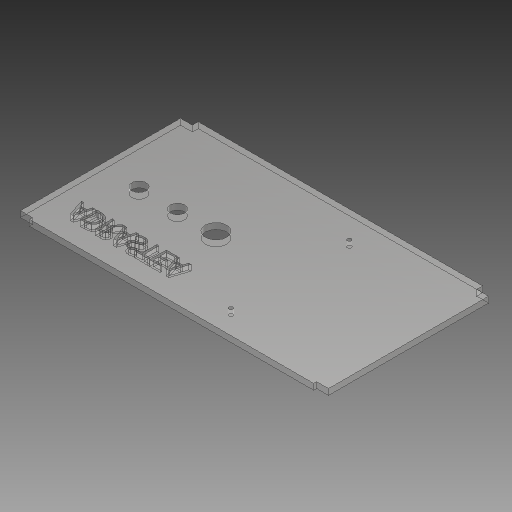
# Autodesk Inventor part: SeitenOben
Saved by Autodesk Inventor 2019 (Build 230136000, 136)
## iProperties
Created: 2018-04-27
Part Number: SeitenOben
Material: Polycarbonate, Clear
Document SubType Name: Modeling
Designer: Phil Erle
Density: 1.2 g/cm^3
Appearance: Polycarbonate - Clear
Author: Phil Erle
Autodesk Inventor part; units mm, degrees
ref_plane "YZ Plane" through (0, 0, 0) normal (1, 0, 0) x (0, 1, 0)
ref_plane "XZ Plane" through (0, 0, 0) normal (0, 1, 0) x (-1, 0, 0)
ref_plane "XY Plane" through (0, 0, 0) normal (0, 0, 1) x (1, 0, 0)
sketch "Sketch1" plane through (0, 0, 0) normal (0, 0, 1) x (1, 0, 0)
  line L0 (-130, 67.5) -> (-130, -67.5)
  line L1 (-130, -67.5) -> (-120, -67.5)
  line L2 (-120, -67.5) -> (-120, -70)
  line L3 (-120, -70) -> (120, -70)
  line L4 (120, -70) -> (120, -67.5)
  line L5 (120, -67.5) -> (130, -67.5)
  line L6 (130, -67.5) -> (130, 67.5)
  line L7 (130, 67.5) -> (120, 67.5)
  line L8 (120, 67.5) -> (120, 72.5)
  line L9 (120, 72.5) -> (-120, 72.5)
  line L10 (-120, 72.5) -> (-120, 67.5)
  line L11 (-130, 67.5) -> (-120, 67.5)
  point P0 (0, 0)
  point P1 (0, 72.5)
  point P2 (130, 0)
  point P3 (-130, 0)
  dimension "d0" = 5
  dimension "d1" = 240
  dimension "d2" = 10
  dimension "d3" = 10
  dimension "d4" = 2.5
  dimension "d5" = 135
  constraints: 24 end point, 8 perpendicular, 7 point on line, 3 midpoint, 1 horizontal alignment, 1 vertical, 1 vertical alignment
  measures "d0" distance of L7.end L8.end
  measures "d1" distance of L8.end L9.end
  measures "d2" distance of L0.start L10.end
  measures "d3" distance of L6.end L7.end
  measures "d4" distance of L3.end L4.end
  measures "d5" distance between parallel lines of L1 L11
extrude "Extrusion1" add sketch "Sketch1" along normal blind 5
sketch "Sketch2" plane through (0, 0, 5) normal (0, 0, 1) x (1, 0, 0)
  point P0 (0, 0)
  point P1 (-65, 0)
  point P2 (-32.5, 0)
  point P3 (-97.5, 0)
  dimension "d8" = 32.5
  dimension "d9" = 32.5
  dimension "d10" = 32.5
  constraints: 3 horizontal alignment
  measures "d8" distance of point (-65, 0) point (-32.5, 0)
  measures "d9" distance of point (0, 0) point (-32.5, 0)
  measures "d10" distance of point (-65, 0) point (-97.5, 0)
hole "Hole1" at (-65, 0, 5) at (-97.5, 0, 5) direction (0, 0, -1) diameter 12 depth 8 tip angle 118
sketch "Sketch3" plane through (0, 0, 5) normal (0, 0, 1) x (1, 0, 0)
  line L0 (30, 50) -> (30, -50) construction
  point P0 (0, 0)
  point P1 (30, 0)
  dimension "d18" = 100
  dimension "d19" = 30
  constraints: 2 coincident, 2 end point, 1 horizontal alignment, 1 midpoint, 1 vertical
  measures "d18" distance of L0.start L0.end
  measures "d19" distance of point (30, 0) point (0, 0)
hole "Hole2" at (30, 50, 5) at (30, -50, 5) direction (0, 0, -1) diameter 3.4 depth 8 tip angle 118 clearance for "Countersunk Flat Head Screw DIN EN ISO 2009" size "M3" standard "DIN"
sketch "Sketch5" plane through (0, 0, 0) normal (0, 0, -1) x (-1, 0, 0)
  line L0 (111.2571, -49) -> (18.7429, -49) construction
  line L1 (18.7429, -49) -> (18.7429, -35) construction
  line L2 (18.7429, -35) -> (111.2571, -35) construction
  line L3 (111.2571, -35) -> (111.2571, -49) construction
  circle A0 centre (65, 0) radius 6 projected
  line L4 (111.3478, -34.7504) -> (106.6282, -48.7504)
  line L5 (106.6282, -48.7504) -> (104.3365, -48.7504)
  line L6 (104.3365, -48.7504) -> (99.6169, -34.7504)
  line L7 (99.6169, -34.7504) -> (101.5796, -34.7504)
  line L8 (101.5796, -34.7504) -> (102.8503, -38.6645)
  line L9 (102.8503, -38.6645) -> (108.1939, -38.6645)
  line L10 (108.1939, -38.6645) -> (109.4645, -34.7504)
  line L11 (109.4645, -34.7504) -> (111.3478, -34.7504)
  line L12 (103.3608, -40.2528) -> (105.5277, -46.8444)
  line L13 (105.5277, -46.8444) -> (107.6833, -40.2528)
  line L14 (107.6833, -40.2528) -> (103.3608, -40.2528)
  spline S0 degree 2 poles (87.2506, -41.7391) (87.2506, -39.8217) (88.8049, -36.7358) (90.1096, -35.8736) knots 0 0 0 1 2 2 2
  spline S1 degree 2 poles (90.1096, -35.8736) (91.176, -35.2042) (93.3657, -34.7504) (95.0675, -34.7504) knots 0 0 0 1 2 2 2
  line L15 (95.0675, -34.7504) -> (98.2895, -34.7504)
  line L16 (98.2895, -34.7504) -> (98.2895, -48.7504)
  line L17 (98.2895, -48.7504) -> (95.1015, -48.7504)
  spline S2 degree 2 poles (95.1015, -48.7504) (93.1274, -48.7504) (90.8811, -48.1605) (90.0869, -47.6386) knots 0 0 0 1 2 2 2
  spline S3 degree 2 poles (90.0869, -47.6386) (88.7368, -46.7423) (87.2506, -43.7812) (87.2506, -41.7391) knots 0 0 0 1 2 2 2
  spline S4 degree 2 poles (89.1906, -41.7617) (89.1906, -43.3728) (90.2571, -45.6532) (91.3122, -46.2998) knots 0 0 0 1 2 2 2
  spline S5 degree 2 poles (91.3122, -46.2998) (92.061, -46.7423) (93.7514, -47.1394) (95.0107, -47.1394) knots 0 0 0 1 2 2 2
  line L18 (95.0107, -47.1394) -> (96.4289, -47.1394)
  line L19 (96.4289, -47.1394) -> (96.4289, -36.3614)
  line L20 (96.4289, -36.3614) -> (95.0107, -36.3614)
  spline S6 degree 2 poles (95.0107, -36.3614) (93.7741, -36.3614) (91.9021, -36.7585) (91.142, -37.2917) knots 0 0 0 1 2 2 2
  spline S7 degree 2 poles (91.142, -37.2917) (90.1663, -37.9498) (89.1906, -40.128) (89.1906, -41.7617) knots 0 0 0 1 2 2 2
  line L21 (74.3965, -34.7504) -> (76.813, -34.7504)
  line L22 (76.813, -34.7504) -> (81.2376, -40.3209)
  line L23 (81.2376, -40.3209) -> (83.3705, -40.3209)
  line L24 (83.3705, -40.3209) -> (83.3705, -34.7504)
  line L25 (83.3705, -34.7504) -> (85.2311, -34.7504)
  line L26 (85.2311, -34.7504) -> (85.2311, -48.7504)
  line L27 (85.2311, -48.7504) -> (81.6234, -48.7504)
  spline S8 degree 2 poles (81.6234, -48.7504) (80.4208, -48.7504) (78.7984, -48.4895) (78.061, -48.013) knots 0 0 0 1 2 2 2
  spline S9 degree 2 poles (78.061, -48.013) (77.3235, -47.5365) (76.4726, -46.0502) (76.4726, -44.9498) knots 0 0 0 1 2 2 2
  spline S10 degree 2 poles (76.4726, -44.9498) (76.4726, -43.4182) (78.0383, -41.342) (79.377, -40.8428) knots 0 0 0 1 2 2 2
  line L28 (79.377, -40.8428) -> (74.3965, -34.7504)
  spline S11 degree 2 poles (78.4127, -44.8023) (78.4127, -45.4149) (78.8438, -46.3566) (79.2976, -46.6629) knots 0 0 0 1 2 2 2
  spline S12 degree 2 poles (79.2976, -46.6629) (79.6947, -46.9238) (80.7498, -47.1394) (81.5213, -47.1394) knots 0 0 0 1 2 2 2
  line L29 (81.5213, -47.1394) -> (83.3705, -47.1394)
  line L30 (83.3705, -47.1394) -> (83.3705, -41.8752)
  line L31 (83.3705, -41.8752) -> (81.7368, -41.8752)
  spline S13 degree 2 poles (81.7368, -41.8752) (80.9313, -41.8752) (79.6493, -42.1588) (79.2068, -42.6013) knots 0 0 0 1 2 2 2
  spline S14 degree 2 poles (79.2068, -42.6013) (78.7984, -42.987) (78.4127, -44.0762) (78.4127, -44.8023) knots 0 0 0 1 2 2 2
  line L32 (74.7935, -34.7504) -> (70.0739, -48.7504)
  line L33 (70.0739, -48.7504) -> (67.7822, -48.7504)
  line L34 (67.7822, -48.7504) -> (63.0626, -34.7504)
  line L35 (63.0626, -34.7504) -> (65.0253, -34.7504)
  line L36 (65.0253, -34.7504) -> (66.296, -38.6645)
  line L37 (66.296, -38.6645) -> (71.6396, -38.6645)
  line L38 (71.6396, -38.6645) -> (72.9102, -34.7504)
  line L39 (72.9102, -34.7504) -> (74.7935, -34.7504)
  line L40 (66.8065, -40.2528) -> (68.9735, -46.8444)
  line L41 (68.9735, -46.8444) -> (71.129, -40.2528)
  line L42 (71.129, -40.2528) -> (66.8065, -40.2528)
  spline S15 degree 2 poles (57.8324, -34.5008) (59.3527, -34.5008) (61.4856, -35.1361) (62.4273, -35.59) knots 0 0 0 1 2 2 2
  line L43 (62.4273, -35.59) -> (62.4273, -37.9271)
  line L44 (62.4273, -37.9271) -> (62.2911, -37.9271)
  spline S16 degree 2 poles (62.2911, -37.9271) (61.3722, -37.0648) (59.0464, -36.1118) (57.9686, -36.1118) knots 0 0 0 1 2 2 2
  spline S17 degree 2 poles (57.9686, -36.1118) (56.4256, -36.1118) (54.8487, -37.3938) (54.8487, -38.4489) knots 0 0 0 1 2 2 2
  spline S18 degree 2 poles (54.8487, -38.4489) (54.8487, -39.2885) (55.6769, -40.3323) (56.5731, -40.5932) knots 0 0 0 1 2 2 2
  spline S19 degree 2 poles (56.5731, -40.5932) (57.2198, -40.7747) (58.2976, -41.0243) (59.1031, -41.2285) knots 0 0 0 1 2 2 2
  spline S20 degree 2 poles (59.1031, -41.2285) (59.8292, -41.4214) (60.9751, -42) (61.4175, -42.4652) knots 0 0 0 1 2 2 2
  spline S21 degree 2 poles (61.4175, -42.4652) (61.8487, -42.9303) (62.3252, -44.1783) (62.3252, -44.9951) knots 0 0 0 1 2 2 2
  spline S22 degree 2 poles (62.3252, -44.9951) (62.3252, -46.6969) (59.6704, -49) (57.6169, -49) knots 0 0 0 1 2 2 2
  spline S23 degree 2 poles (57.6169, -49) (56.437, -49) (54.3495, -48.5348) (53.4532, -48.0924) knots 0 0 0 1 2 2 2
  line L45 (53.4532, -48.0924) -> (53.4532, -45.8687)
  line L46 (53.4532, -45.8687) -> (53.5893, -45.8687)
  spline S24 degree 2 poles (53.5893, -45.8687) (54.2587, -46.4814) (56.3462, -47.389) (57.4921, -47.389) knots 0 0 0 1 2 2 2
  spline S25 degree 2 poles (57.4921, -47.389) (58.7854, -47.389) (60.3851, -46.175) (60.3851, -45.188) knots 0 0 0 1 2 2 2
  spline S26 degree 2 poles (60.3851, -45.188) (60.3851, -44.3031) (59.4435, -43.248) (58.5585, -43.0097) knots 0 0 0 1 2 2 2
  spline S27 degree 2 poles (58.5585, -43.0097) (57.9686, -42.8509) (56.2555, -42.4425) (55.6882, -42.2723) knots 0 0 0 1 2 2 2
  spline S28 degree 2 poles (55.6882, -42.2723) (54.2474, -41.8298) (52.9086, -40.0486) (52.9086, -38.7439) knots 0 0 0 1 2 2 2
  spline S29 degree 2 poles (52.9086, -38.7439) (52.9086, -37.9157) (53.578, -36.3274) (54.1793, -35.7715) knots 0 0 0 1 2 2 2
  spline S30 degree 2 poles (54.1793, -35.7715) (54.8487, -35.1588) (56.5504, -34.5008) (57.8324, -34.5008) knots 0 0 0 1 2 2 2
  line L47 (47.7465, -34.7504) -> (47.7465, -47.094)
  line L48 (47.7465, -47.094) -> (52.4435, -47.094)
  line L49 (52.4435, -47.094) -> (52.4435, -48.7504)
  line L50 (52.4435, -48.7504) -> (41.189, -48.7504)
  line L51 (41.189, -48.7504) -> (41.189, -47.094)
  line L52 (41.189, -47.094) -> (45.8859, -47.094)
  line L53 (45.8859, -47.094) -> (45.8859, -34.7504)
  line L54 (45.8859, -34.7504) -> (47.7465, -34.7504)
  line L55 (39.7709, -34.7504) -> (39.7709, -48.7504)
  line L56 (39.7709, -48.7504) -> (31.0123, -48.7504)
  line L57 (31.0123, -48.7504) -> (31.0123, -47.094)
  line L58 (31.0123, -47.094) -> (37.9102, -47.094)
  line L59 (37.9102, -47.094) -> (37.9102, -43.2593)
  line L60 (37.9102, -43.2593) -> (31.4775, -43.2593)
  line L61 (31.4775, -43.2593) -> (31.4775, -41.6029)
  line L62 (31.4775, -41.6029) -> (37.9102, -41.6029)
  line L63 (37.9102, -41.6029) -> (37.9102, -36.4068)
  line L64 (37.9102, -36.4068) -> (31.0123, -36.4068)
  line L65 (31.0123, -36.4068) -> (31.0123, -34.7504)
  line L66 (31.0123, -34.7504) -> (39.7709, -34.7504)
  line L67 (30.4791, -34.7504) -> (25.7595, -48.7504)
  line L68 (25.7595, -48.7504) -> (23.4678, -48.7504)
  line L69 (23.4678, -48.7504) -> (18.7482, -34.7504)
  line L70 (18.7482, -34.7504) -> (20.7109, -34.7504)
  line L71 (20.7109, -34.7504) -> (21.9816, -38.6645)
  line L72 (21.9816, -38.6645) -> (27.3252, -38.6645)
  line L73 (27.3252, -38.6645) -> (28.5958, -34.7504)
  line L74 (28.5958, -34.7504) -> (30.4791, -34.7504)
  line L75 (22.4921, -40.2528) -> (24.659, -46.8444)
  line L76 (24.659, -46.8444) -> (26.8146, -40.2528)
  line L77 (26.8146, -40.2528) -> (22.4921, -40.2528)
  point P0 (0, 0)
  point P1 (65, -49)
  dimension "d31" = 35
  dimension "d32" = 14
  constraints: 1 midpoint, 1 vertical alignment, 2 other
  measures "d31" distance from line of A0.centre L2
  measures "d32" distance between parallel lines of L0 L2
extrude "Extrusion3" cut sketch "Sketch5" against normal blind 10 contours L4 L5 L6 L7 L8 L9 L10 L11 | S0 S1 L15 L16 L17 S2 S3 | L21 L32 L28 | L28 L32 L33 L34 L35 L36 L37 L38 L39 | L21 L22 L23 L24 L25 L26 L27 S8 S9 S10 L28 L32 | S15 L43 L44 S16 S17 S18 S19 S20 S21 S22 S23 L45 L46 S24 S25 S26 S27 S28 S29 S30 | L47 L48 L49 L50 L51 L52 L53 L54 | L55 L56 L57 L58 L59 L60 L61 L62 L63 L64 L65 L66 | L67 L68 L69 L70 L71 L72 L73 L74
sketch "Sketch6" plane through (0, 0, 5) normal (0, 0, 1) x (1, 0, 0)
  point P0 (0, 0)
  point P1 (-32.5, 0)
  dimension "d35" = 32.5
  constraints: 1 horizontal alignment
  measures "d35" distance of point (0, 0) point (-32.5, 0)
hole "Hole3" at (-32.5, 0, 5) direction (0, 0, -1) diameter 18 depth 8 tip angle 118
equation "\"d9\" = d8"
equation "\"d10\" = d8"
body "Solid1"
